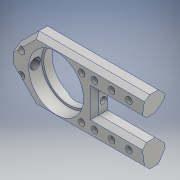
# Autodesk Inventor part: mirrormountv3
Saved by Autodesk Inventor 2017 SP1 (Build 210196100, 196)
## iProperties
Created: 2018-05-21
Part Number: mirrormountv3
Material: Aluminum 6061
Document SubType Name: Modeling
Designer: Sam
Mass: 2.53126 g
Surface Area: 13.1979 cm^2
Volume: 0.937504 cm^3
Density: 2.7 g/cm^3
Appearance: Aluminum - Flat
Author: Sam
Autodesk Inventor part; units mm, degrees
ref_plane "YZ Plane" through (0, 0, 0) normal (1, 0, 0) x (0, 1, 0)
ref_plane "XZ Plane" through (0, 0, 0) normal (0, 1, 0) x (-1, 0, 0)
ref_plane "XY Plane" through (0, 0, 0) normal (0, 0, 1) x (1, 0, 0)
sketch "Sketch1" plane through (0, 0, 0) normal (0, 1, 0) x (-1, 0, 0)
  line L0 (0, 0) -> (65, 0)
  line L1 (65, 0) -> (65, -15)
  line L2 (65, -15) -> (0, -15)
  line L3 (0, -15) -> (0, 0)
  dimension "d0" = 65
  dimension "d1" = 15
  constraints: 8 end point, 2 parallel, 1 horizontal, 1 perpendicular
  measures "d0" distance of L1.end L2.end
  measures "d1" distance of L0.end L1.end
extrude "Extrusion1" add sketch "Sketch1" along normal blind 6
sketch "Sketch2" plane through (0, 0, 0) normal (0, -1, 0) x (1, 0, 0)
  line L0 (0, 0) -> (0, -15) projected
  circle A0 centre (0, -7.5) radius 35
  dimension "d4" = 70
  constraints: 1 centre point, 1 midpoint
  measures "d4" diameter of A0
extrude "Extrusion2" cut sketch "Sketch2" against normal blind 6
sketch "Sketch3" plane through (0, 0, 0) normal (0, -1, 0) x (1, 0, 0)
  circle A0 centre (-55, -7.5591) radius 6.4
  arc A1 (-34.187, 0) -> (-34.187, -15) centre (0, -7.5) ccw projected
  point P0 (0, 0)
  dimension "d7" = 12.8
  dimension "d10" = 55
  constraints: 1 centre point
  measures "d7" diameter of A0
  measures "d10" distance of A1.centre A0.centre
extrude "Extrusion3" cut sketch "Sketch3" against normal blind 4
sketch "Sketch4" plane through (-55, 4, -7.5591) normal (0, -1, 0) x (1, 0, 0)
  circle A0 centre (0, 0) radius 5.9
  point P0 (55, 7.5591)
  dimension "d11" = 11.8
  constraints: 1 centre point
  measures "d11" diameter of A0
extrude "Extrusion4" cut sketch "Sketch4" against normal blind 4
sketch "Sketch5" plane through (-65, 0, -15) normal (-1, 0, 0) x (0, 0, 1)
  line L0 (15, 0) -> (0, 0) projected
  point P0 (7.5, 2.5)
  dimension "d21" = 2.5
  measures "d21" distance from line of point (7.5, 2.5) L0
hole "Hole1" at (-65, 2.5, -7.5) direction (1, 0, 0) diameter 2.459 depth 8.8 tip angle 118 thread size "M3x0.5" class "6H" standard "ISO Metric profile"
sketch "Sketch6" plane through (0, 0, 0) normal (0, -1, 0) x (1, 0, 0)
  line L0 (-34, -10) -> (-46, -10)
  line L1 (-46, -10) -> (-46, -5)
  line L2 (-46, -5) -> (-34, -5)
  line L3 (-34, -5) -> (-34, -10)
  point P0 (0, 0)
  dimension "d22" = 12
  dimension "d23" = 5
  constraints: 8 end point, 2 parallel, 1 horizontal, 1 perpendicular
  measures "d22" distance of L1.end L2.end
  measures "d23" distance of L0.end L1.end
extrude "Extrusion5" cut sketch "Sketch6" against normal blind 6
chamfer "Chamfer1" distance 5 angle 45 2 edges at (-65, 3, -15) (-65, 3, 0)
chamfer "Chamfer2" distance 2 angle 45 10 edges at (-47.0935, 6, -15) (-47.0935, 6, 0) (-40.4553, 6, -5) (-46, 6, -7.5) (-40.4553, 6, -10) (-47.0935, 0, -15) (-47.0935, 0, 0) (-40.4553, 0, -10) (-46, 0, -7.5) (-40.4553, 0, -5)
sketch "Sketch7" plane through (0, 0, 0) normal (0, -1, 0) x (1, 0, 0)
  point P0 (0, 0)
  point P1 (-63, -5)
  point P2 (-63, -10)
hole "Hole2" at (-63, 0, -5) at (-63, 0, -10) direction (0, 1, 0) diameter 1.5 end through all
sketch "Sketch8" plane through (0, 0, 0) normal (0, -1, 0) x (1, 0, 0)
  point P0 (0, 0)
  point P1 (-38, -2.5)
  point P2 (-42, -2.5)
  point P3 (-46, -2.5)
  point P4 (-38, -12.5)
  point P5 (-42, -12.5)
  point P6 (-46, -12.5)
hole "Hole3" at (-38, 0, -2.5) at (-42, 0, -2.5) at (-46, 0, -2.5) at (-38, 0, -12.5) at (-42, 0, -12.5) at (-46, 0, -12.5) direction (0, 1, 0) diameter 1.5 end through all
chamfer "Chamfer3" distance 1 angle 45 1 edges at (-65, 0, -7.5)
chamfer "Chamfer4" distance 1 angle 45 3 edges at (-65, 6, -7.5) (-65, 3.5, -5) (-65, 3.5, -10)
sketch "Sketch9" plane through (0, 0, 0) normal (0, -1, 0) x (1, 0, 0)
  line L0 (-33.161, -16.171) -> (-65.6535, -16.171)
  line L1 (-65.6535, -16.171) -> (-65.6535, 0.5544)
  line L2 (-65.6535, 0.5544) -> (-33.161, 0.5544)
  line L3 (-33.161, 0.5544) -> (-33.161, -16.171)
  point P0 (0, 0)
  constraints: 8 end point, 2 parallel, 1 horizontal, 1 perpendicular
extrude "Extrusion6" cut sketch "Sketch9" against normal blind 1
chamfer "Chamfer5" distance 1 angle 45 2 edges at (-62.6464, 1, -12.3536) (-62.6464, 1, -2.6464)
sketch "Sketch10" plane through (0, 1, 0) normal (0, -1, 0) x (1, 0, 0)
  point P0 (0, 0)
  point P1 (-49, -12.5)
  point P2 (-49, -2.5)
hole "Hole4" at (-49, 1, -12.5) at (-49, 1, -2.5) direction (0, 1, 0) diameter 1.5 end through all
sketch "Sketch11" plane through (-46, 2, -10) normal (1, 0, 0) x (0, 0, -1)
  point P0 (-10, -2)
  point P1 (-2.5, 1)
hole "Hole5" at (-46, 3, -7.5) direction (-1, 0, 0) diameter 1.5 end through all
body "Solid1"
